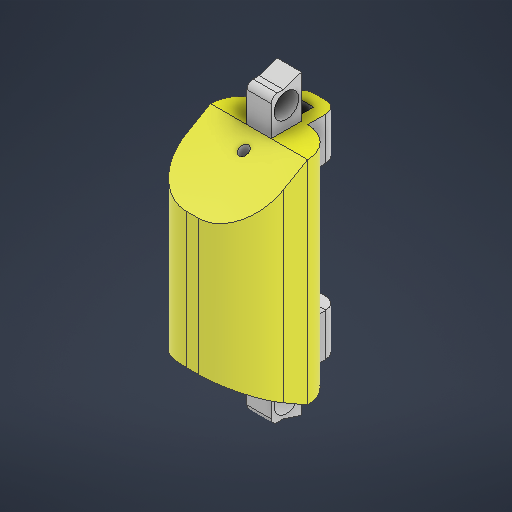
# Autodesk Inventor part: FingerMiddle
Saved by Autodesk Inventor 2026 (Build 300175050, 175E)
## iProperties
Created: 2026-05-22
Part Number: FingerMiddle
Material: Generic
Document SubType Name: Modeling
Designer: SaiAn
Density: 1 g/cm^3
Appearance: Default
Author: SaiAn
Autodesk Inventor part; units mm, degrees
ref_plane "YZ Plane" through (0, 0, 0) normal (1, 0, 0) x (0, 1, 0)
ref_plane "XZ Plane" through (0, 0, 0) normal (0, 1, 0) x (-1, 0, 0)
ref_plane "XY Plane" through (0, 0, 0) normal (0, 0, 1) x (1, 0, 0)
sketch "Sketch3" plane through (0, 0, 0) normal (0, 0, 1) x (1, 0, 0)
  line L0 (0, 0) -> (16, 0)
  line L1 (16, 0) -> (16, 35)
  line L2 (16, 35) -> (0, 35)
  line L3 (0, 35) -> (0, 0)
  dimension "d0" = 16
  dimension "d1" = 35
  constraints: 8 end point, 2 parallel, 1 horizontal, 1 perpendicular
  measures "d0" distance of L2.end L1.end
  measures "d1" distance of L1.end L0.end
extrude "Extrusion1" add sketch "Sketch3" along normal blind 16
fillet "Fillet1" radius 7 2 edges at (16, 17.5, 16) (0, 17.5, 16)
fillet "Fillet2" radius 5 2 edges at (16, 17.5, 0) (0, 17.5, 0)
sketch "Sketch4" plane through (16, 0, 9) normal (1, 0, 0) x (0, 0, -1)
  line L0 (4, 35) -> (0, 35) projected
  line L1 (4, 35) -> (-7, 28.6491)
  line L2 (-7, 35) -> (-7, 0) projected
  line L3 (4, 35) -> (16.7017, 35) construction
  line L4 (-7, 28.6491) -> (-7, 35)
  line L5 (-7, 35) -> (4, 35)
  line L6 (4, 0) -> (0, 0) projected
  line L7 (4, 0) -> (-7, 6.3509)
  line L8 (4, 0) -> (16.7017, 0) construction
  line L9 (-7, 6.3509) -> (-7, 0)
  line L10 (-7, 0) -> (4, 0)
  point P0 (9, 0)
  point P1 (-7, 0)
  point P2 (0, 0)
  dimension "d6" = 150
  dimension "d7" = 150
  constraints: 16 end point, 3 point on line, 2 equal length, 2 horizontal, 2 perpendicular, 1 collinear
  measures "d6" angle of L1 L3
  measures "d7" angle of L8 L7
extrude "Extrusion2" cut sketch "Sketch4" against normal through all
sketch "Sketch5" plane through (5, 35, 0) normal (0, 1, 0) x (1, 0, 0)
  line L0 (-5, -9) -> (-5, -5) projected
  line L1 (0, 0) -> (6, 0) projected
  line L2 (5, 0) -> (1, 0)
  line L3 (1, 0) -> (1, -5)
  line L4 (1, -5) -> (5, -5)
  line L5 (5, -5) -> (5, 0)
  line L6 (1, 0) -> (5, 0)
  point P0 (-5, 0)
  dimension "d47" = 4
  constraints: 10 end point, 2 parallel, 1 collinear, 1 horizontal, 1 perpendicular, 1 point on line
  measures "d47" distance of L4.end L3.end
extrude "Extrusion3" add sketch "Sketch5" along normal blind 6
sketch "Sketch11" plane through (0, 0, 0) normal (0, 0, -1) x (-1, 0, 0)
  line L0 (-11, 0) -> (-11, 35) projected
  line L1 (-9, 28.6491) -> (-9, 6.3509) projected
  line L2 (-11, 0) -> (-9, 0)
  line L3 (-9, 0) -> (-9, 7)
  line L4 (-9, 7) -> (-11, 7)
  line L5 (-11, 7) -> (-11, 0)
  line L6 (-5, 0) -> (-7, 0)
  line L7 (-7, 0) -> (-7, 7)
  line L8 (-7, 7) -> (-5, 7)
  line L9 (-5, 7) -> (-5, 0)
  line L10 (-11, 35) -> (-9, 35)
  line L11 (-9, 35) -> (-9, 28)
  line L12 (-9, 28) -> (-11, 28)
  line L13 (-11, 28) -> (-11, 35)
  line L14 (-5, 35) -> (-7, 35)
  line L15 (-7, 35) -> (-7, 28)
  line L16 (-7, 28) -> (-5, 28)
  line L17 (-5, 28) -> (-5, 35)
  point P0 (0, 0)
  point P1 (-9, 6.3509)
  point P2 (-11, 28)
  dimension "d32" = 7
  dimension "d33" = 2
  dimension "d34" = 7
  dimension "d35" = 7
  dimension "d36" = 7
  constraints: 32 end point, 8 parallel, 4 horizontal, 4 perpendicular, 4 point on line
  measures "d32" distance of L3.end L2.end
  measures "d33" distance of L7.end L8.end
  measures "d34" distance of L6.end L7.end
  measures "d35" distance of L10.end L11.end
  measures "d36" distance of L15.end L14.end
extrude "Extrusion9" add sketch "Sketch11" along normal blind 3 contours L0 L4 L1 L3 L2 | L0 L10 L11 L1 L12 | L6 L7 L8 L9 | L17 L16 L15 L14
sketch "Sketch12" plane through (0, 0, -3) normal (0, 0, -1) x (-1, 0, 0)
  line L0 (-9, 35) -> (-11, 35) projected
  line L1 (-5, 28) -> (-7, 28) projected
  line L2 (-11, 35) -> (-5, 35)
  line L3 (-5, 35) -> (-5, 28)
  line L4 (-5, 28) -> (-11, 28)
  line L5 (-11, 28) -> (-11, 35)
  line L6 (-11, 0) -> (-16, 0) projected
  line L7 (-11, 0) -> (-5, 0)
  line L8 (-5, 0) -> (-5, 7.0241)
  line L9 (-5, 7.0241) -> (-11, 7.0241)
  line L10 (-11, 7.0241) -> (-11, 0)
  point P0 (0, 0)
  point P1 (-5, -5)
  point P2 (-11, 2)
  constraints: 16 end point, 4 parallel, 2 horizontal, 2 perpendicular, 2 point on line
extrude "Extrusion10" add sketch "Sketch12" along normal blind 2
sketch "Sketch13" plane through (0, 0, 5) normal (0, -1, 0) x (1, 0, 0)
  circle A0 centre (8, 2.5) radius 0.75
  point P0 (0, -5)
  dimension "d42" = 1.5
  constraints: 1 centre point
  measures "d42" diameter of A0
extrude "Extrusion11" cut sketch "Sketch13" against normal through all
fillet "Fillet4" radius 2 4 edges at (11, 31.5, -5) (5, 31.5, -5) (5, 3.5121, -5) (11, 3.5121, -5)
sketch "Sketch14" plane through (10, 35, 5) normal (1, 0, 0) x (0, 0, -1)
  circle A0 centre (2.5, 3.5) radius 2.025
  line L0 (0, 6) -> (5, 6) projected
  point P0 (5, -35)
  dimension "d48" = 4.05
  dimension "d59" = 2.5
  constraints: 1 centre point
  measures "d48" diameter of A0
  measures "d59" distance from line of L0 A0.centre
extrude "Extrusion12" cut sketch "Sketch14" against normal blind 5
sketch "Sketch15" plane through (0, 0, 5) normal (0, -1, 0) x (1, 0, 0)
  line L0 (10, -5) -> (10, 0) projected
  line L1 (10, 0) -> (6, 0)
  line L2 (6, 0) -> (6, -5)
  line L3 (6, -5) -> (10, -5)
  line L4 (10, -5) -> (10, 0)
  point P0 (0, -5)
  point P1 (10, -0.475)
  point P2 (6, -0.475)
  dimension "d60" = 5
  dimension "d61" = 4
  constraints: 8 end point, 2 parallel, 1 horizontal, 1 perpendicular
  measures "d60" distance of L1.end L2.end
  measures "d61" distance of L2.end L3.end
extrude "Extrusion13" add sketch "Sketch15" along normal blind 6
sketch "Sketch16" plane through (10, 0, 5) normal (1, 0, 0) x (0, 0, -1)
  circle A0 centre (2.5, -3.5) radius 2.025
  line L0 (5, -6) -> (0, -6) projected
  point P0 (5, 0)
  dimension "d54" = 4.05
  dimension "d58" = 2.5
  constraints: 1 centre point
  measures "d54" diameter of A0
  measures "d58" distance from line of L0 A0.centre
extrude "Extrusion14" cut sketch "Sketch16" against normal blind 5
fillet "Fillet7" radius 1 1 edges at (8, -6, 5)
sketch "Sketch17" plane through (0, -6, 5) normal (0, -1, 0) x (1, 0, 0)
  line L0 (6, -5) -> (10, -5) projected
  line L1 (6, -4.525) -> (6, -0.475) projected
  line L2 (10, -5) -> (6, -5)
  line L3 (6, -5) -> (6, -2)
  line L4 (6, -2) -> (10, -2)
  line L5 (10, -2) -> (10, -5)
  point P0 (0, -5)
  dimension "d63" = 3
  constraints: 8 end point, 2 parallel, 1 horizontal, 1 perpendicular, 1 point on line
  measures "d63" distance of L2.end L3.end
extrude "Extrusion15" add sketch "Sketch17" along normal blind 1
fillet "Fillet8" radius 1 1 edges at (8, 41, 5)
sketch "Sketch18" plane through (5, 41, 0) normal (0, 1, 0) x (1, 0, 0)
  line L0 (1, -3) -> (5, -3) projected
  line L1 (1, -5) -> (1, 0) projected
  line L2 (5, -3) -> (1, -3)
  line L3 (1, -3) -> (1, 0)
  line L4 (1, 0) -> (5, 0)
  line L5 (5, 0) -> (5, -3)
  point P0 (-5, 0)
  constraints: 8 end point, 2 parallel, 1 horizontal, 1 perpendicular
extrude "Extrusion16" add sketch "Sketch18" along normal blind 1
sketch "Sketch19" plane through (6, 0, 0) normal (-1, 0, 0) x (0, 0, 1)
  line L0 (3, -6) -> (3, -7) projected
  line L1 (0, 0) -> (0, -7) projected
  line L2 (3, -6) -> (0, -7)
  line L3 (0, -7) -> (3, -7)
  line L4 (3, -7) -> (3, -6)
  constraints: 6 end point, 2 perpendicular
extrude "Extrusion17" cut sketch "Sketch19" against normal through all
sketch "Sketch20" plane through (6, 35, 0) normal (-1, 0, 0) x (0, 0, 1)
  line L0 (4, 6) -> (3, 6) projected
  line L1 (0, 0) -> (0, 7) projected
  line L2 (3, 6) -> (0, 7)
  line L3 (0, 7) -> (3, 7)
  line L4 (3, 7) -> (3, 6)
  point P0 (0, -35)
  constraints: 6 end point, 2 perpendicular
extrude "Extrusion18" cut sketch "Sketch20" against normal through all
body "Solid1"
